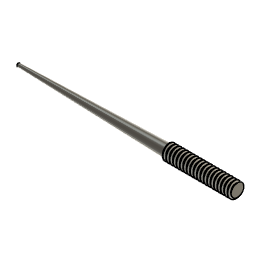
multi_tip_design (Autodesk Fusion 360 archive; units mm, degrees)
design "Single tip design"
Autodesk Fusion 360 part; units mm, degrees
sketch "Sketch1" plane through (0, 0, 0) normal (0, 1, 0) x (1, 0, 0)
  line L0 (0, -22.8363) -> (0, 25.9446) construction
  line L1 (0, 0) -> (0, -1.3335)
  line L2 (0, -1.3335) -> (-35.0388, -0.3701)
  line L3 (0, -1.3335) -> (35.052, -1.3335) construction
  line L4 (0, 0) -> (-35.0388, 0)
  line L5 (-35.0388, 0) -> (-35.0388, -0.3701)
  line L6 (0, 0) -> (15.748, 0)
  line L7 (15.748, 0) -> (15.748, -1.651)
  line L8 (15.748, -1.651) -> (0, -1.651)
  line L9 (0, -1.3335) -> (0, -1.651)
  dimension "d6" = 1.3335
  dimension "d7" = 178.425
  dimension "d8" = 35.052
  dimension "d9" = 15.748
  dimension "d10" = 1.651
  constraint coincident L1.start L4.start
  constraint parallel L0 L1
  constraint horizontal L3
  constraint perpendicular L0 L4
  constraint parallel L0 L5
  constraint perpendicular L0 L6
  constraint perpendicular L3 L7
  constraint coincident L0 L8.end
  constraint perpendicular L0 L8
  constraint perpendicular L8 L9
  measures "d6" distance of L1.start L1.end
  measures "d7" angle of L2 L3
  measures "d8" distance of L1.end L2.end
  measures "d9" distance of L1.start L6.end
  measures "d10" distance of L6.end L7.end
revolve "Revolve1" add sketch "Sketch1" angle 360 about axis through (0, 0, 0) along (-1, 0, 0)
thread "Thread1" "ANSI Unified Screw Threads 0.138(#6) 6-32 UNC 2A" major diameter 3.4087 minor diameter 2.54 pitch 0.7937 angle 60 modelled right hand crest width 0.1226 on face at (10.4987, -0.0823, 1.6489) crest through (15.9464, 0, 1.7043)
equation "d6 = ( ( 0.105 / 2 ) * 1 in )"
